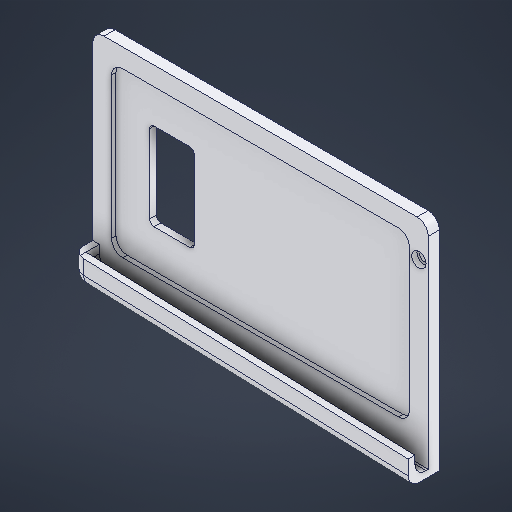
# Autodesk Inventor part: panel-suport
Saved by Autodesk Inventor 2026.2 (Build 302298010, 298A)
## iProperties
Created: 2026-04-07
Part Number: panel-suport
Material: Plástico PET
Document SubType Name: Modeling
Designer: Aluno
Density: 1.541 g/cm^3
Appearance: PTFE
Author: Aluno
Autodesk Inventor part; units mm, degrees
ref_plane "YZ Plane" through (0, 0, 0) normal (1, 0, 0) x (0, 1, 0)
ref_plane "XZ Plane" through (0, 0, 0) normal (0, 1, 0) x (-1, 0, 0)
ref_plane "XY Plane" through (0, 0, 0) normal (0, 0, 1) x (1, 0, 0)
sketch "Sketch1" plane through (0, 0, 0) normal (0, 0, 1) x (1, 0, 0)
  line L0 (-75, 45) -> (75, 45)
  line L1 (75, 45) -> (75, -45)
  line L2 (75, -45) -> (-75, -45)
  line L3 (-75, -45) -> (-75, 45)
  line L4 (-75, 45) -> (75, -45) construction
  line L5 (75, 45) -> (-75, -45) construction
  point P0 (0, 0)
  dimension "d0" = 150
  dimension "d1" = 90
  constraints: 12 end point, 2 midpoint, 2 parallel, 1 horizontal, 1 perpendicular
  measures "d0" distance of L1.end L2.end
  measures "d1" distance of L0.end L1.end
extrude "Extrusion1" add sketch "Sketch1" along normal blind 5
fillet "Fillet1" radius 5 2 edges at (-75, 45, 2.5) (75, 45, 2.5)
sketch "Sketch2" plane through (0, 0, 5) normal (0, 0, 1) x (1, 0, 0)
  line L0 (-61.6, -36.6) -> (61.6, -36.6)
  line L1 (66.6, -31.6) -> (66.6, 31.6)
  line L2 (61.6, 36.6) -> (-61.6, 36.6)
  line L3 (-66.6, 31.6) -> (-66.6, -31.6)
  line L4 (-66.6, -36.6) -> (66.6, 36.6) construction
  line L5 (66.6, -36.6) -> (-66.6, 36.6) construction
  arc A0 (-61.6, 36.6) -> (-66.6, 31.6) centre (-61.6, 31.6) ccw
  arc A1 (-66.6, -31.6) -> (-61.6, -36.6) centre (-61.6, -31.6) ccw
  arc A2 (61.6, -36.6) -> (66.6, -31.6) centre (61.6, -31.6) ccw
  arc A3 (66.6, 31.6) -> (61.6, 36.6) centre (61.6, 31.6) ccw
  point P0 (0, 0)
  dimension "d5" = 133.2
  dimension "d6" = 73.2
  dimension "d9" = 5
  constraints: 12 end point, 8 point on circle, 8 point on line, 8 tangent, 4 centre point, 3 equal radius, 2 midpoint, 2 parallel, 1 horizontal, 1 perpendicular
  measures "d5" distance of L5.end L4.end
  measures "d6" distance of L5.start L4.end
  measures "d9" radius of A0
extrude "Extrusion2" cut sketch "Sketch2" against normal blind 2
sketch "Sketch3" plane through (0, 0, 5) normal (0, 0, 1) x (1, 0, 0)
  line L0 (66.6, 31.6) -> (66.6, -31.6) projected
  line L1 (66.6, 0) -> (75, 0) construction
  line L2 (75, -45) -> (75, 40) projected
  line L3 (70.8, 0) -> (70.8, 28.8336) construction
  circle A0 centre (70.8, 28.8336) radius 3.25
  point P0 (0, 0)
  point P1 (75, -40)
  dimension "d10" = 6.5
  constraints: 4 end point, 2 midpoint, 1 centre point, 1 coincident, 1 point on line, 1 vertical
  measures "d10" diameter of A0
extrude "Extrusion3" cut sketch "Sketch3" against normal blind 2.4
sketch "Sketch4" plane through (70.8, 28.8336, 2.6) normal (0, 0, 1) x (1, 0, 0)
  circle A0 centre (0, 0) radius 2
  point P0 (-70.8, -28.8336)
  dimension "d13" = 4
  constraints: 1 centre point
  measures "d13" diameter of A0
extrude "Extrusion4" cut sketch "Sketch4" against normal blind 15
sketch "Sketch7" plane through (0, 0, 3) normal (0, 0, 1) x (1, 0, 0)
  line L0 (-66.6, -31.6) -> (-66.6, 31.6) projected
  line L1 (-66.6, 0.4) -> (-51.6, 0.4) construction
  line L2 (61.6, -36.6) -> (-61.6, -36.6) projected
  line L3 (-51.6, -36.6) -> (-51.6, -19.6) construction
  line L4 (-51.6, -36.6) -> (-34.6, -36.6) construction
  line L5 (-66.6, 19.9067) -> (-31.6, 19.9067) construction
  line L6 (-31.6, -17.6) -> (-31.6, 19.4) construction
  line L7 (-31.6, -36.6) -> (5.4, -36.6) construction
  line L8 (-49.6, -19.6) -> (-33.6, -19.6)
  line L9 (-31.6, -19.6) -> (-31.6, 17.4)
  line L10 (-33.6, 19.4) -> (-49.6, 19.4)
  line L11 (-51.6, 17.4) -> (-51.6, -17.6)
  arc A0 (-49.6, 19.4) -> (-51.6, 17.4) centre (-49.6, 17.4) ccw
  arc A1 (-31.6, 17.4) -> (-33.6, 19.4) centre (-33.6, 17.4) ccw
  arc A2 (-33.6, -19.6) -> (-31.6, -17.6) centre (-33.6, -17.6) ccw
  arc A3 (-51.6, -17.6) -> (-49.6, -19.6) centre (-49.6, -17.6) ccw
  point P0 (0, 0)
  point P1 (-67, -23.834)
  point P2 (-31.6, -17.6)
  dimension "d30" = 17
  dimension "d31" = 90
  dimension "d34" = 56
  dimension "d35" = 90
  dimension "d36" = 15
  dimension "d37" = 35
  dimension "d38" = 2
  constraints: 20 end point, 8 point on circle, 8 point on line, 8 tangent, 5 horizontal, 4 centre point, 4 perpendicular, 3 equal radius, 2 parallel, 1 vertical, 3 other
  measures "d30" distance of L3.start L3.end
  measures "d31" angle of L4 L3
  measures "d34" distance of L7.start L6.end
  measures "d35" angle of L7 L6
  measures "d38" radius of A0
extrude "Extrusion6" cut sketch "Sketch7" against normal blind 8.25
sketch "Esboço13" plane through (0, 0, 5) normal (0, 0, 1) x (1, 0, 0)
  line L0 (-75, -45) -> (75, -45) projected
  line L1 (-75, -45) -> (75, -50.2381)
  line L2 (75, -45) -> (75, -50.2381) construction
  line L3 (-75, -45) -> (-75, -48)
  line L4 (-75, -48) -> (75, -53.2381)
  line L5 (75, -50.2381) -> (75, -53.2381)
  point P0 (0, 0)
  dimension "d56" = 2
  dimension "d57" = 3
  constraints: 10 end point, 3 vertical, 1 parallel
  measures "d56" angle of L0 L1
  measures "d57" distance of L0.start L3.end
extrude "Extrusão12" add sketch "Esboço13" along normal blind 6
sketch "Esboço14" plane through (-75, -45, 0) normal (0, -1, 0) x (1, 0, 0)
  line L0 (0, 5) -> (150, 5) projected
  line L1 (0, 0) -> (150, 0)
  line L2 (150, 0) -> (150, 5)
  line L3 (150, 5) -> (0, 5)
  line L4 (0, 5) -> (0, 0)
  point P0 (75, 0)
  constraints: 8 end point, 2 parallel, 1 horizontal, 1 perpendicular
extrude "Extrusão13" add sketch "Esboço14" along normal up to surface surface through (-75, -48, 5) normal (-0.0348995, -0.9993908, 0)
sketch "Esboço16" plane through (0, 0, 5) normal (0, 0, 1) x (1, 0, 0)
  line L0 (61.6, -36.6) -> (-61.6, -36.6) projected
  line L1 (-61.6, -36.6) -> (-72, -36.6) construction
  line L2 (-75, -45) -> (-75, -48) projected
  line L3 (-75, -45) -> (-75, -36.6)
  line L4 (-75, 40) -> (-75, -45) projected
  line L5 (-72, -45.1048) -> (-72, -36.6)
  line L6 (-72, -36.6) -> (-75, -36.6)
  line L7 (-75, -45) -> (-72, -45.1048)
  line L8 (75, -50.2381) -> (-75, -45) projected
  point P0 (0, 0)
  dimension "d63" = 3
  constraints: 10 end point, 3 collinear, 2 horizontal, 1 point on line
  measures "d63" distance between parallel lines of L3 L5
extrude "Extrusão14" add sketch "Esboço16" along normal up to surface (6 mm away)
sketch "Esboço17" plane through (0, 0, 11) normal (0, 0, 1) x (1, 0, 0)
  line L0 (-75, -36.6) -> (-72, -36.6) projected
  line L1 (-72, -36.6) -> (75, -41.7334)
  line L2 (75, -50.2381) -> (-72, -45.1048) projected
  line L3 (75, 40) -> (75, -53.2381) projected
  line L4 (75, -53.2381) -> (75, -41.7334)
  line L5 (-72, -36.6) -> (-72, -45.1048) projected
  line L6 (-72, -36.6) -> (-75, -36.6)
  line L7 (-75, -48) -> (-75, -36.6) projected
  line L8 (-75, -36.6) -> (-75, -48)
  line L9 (-75, -48) -> (75, -53.2381)
  point P0 (0, 0)
  constraints: 10 end point, 2 equal length, 1 perpendicular, 1 vertical
extrude "Extrusão15" add sketch "Esboço17" along normal blind 3
fillet "Arredondamento3" radius 5 1 edges at (0, -50.6191, 14)
fillet "Arredondamento4" radius 5 2 edges at (1.5, -47.6714, 11) (-72, -45.1048, 8)
fillet "Arredondamento5" radius 5 3 edges at (-75, -48, 4.5) (-75, -39.7985, 14) (-75, -46.5346, 12.5355)
body "Solid1"
